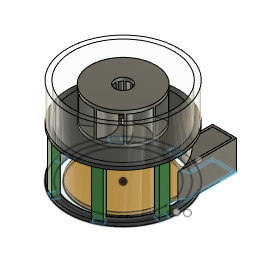
Impeller Design v6 (Autodesk Fusion 360 design; units mm, degrees)
Autodesk Fusion 360 part; units mm, degrees
sketch "Skizze1" plane through (0, 0, 0) normal (0, 0, 1) x (1, 0, 0)
  circle A0 centre (0, 0) radius 100
  circle A1 centre (0, 0) radius 25
  dimension "d1" = 200
  dimension "d2" = 50
  constraint coincident A0.centre A1.centre
  constraint concentric A0 A1
  measures "d1" diameter of A0
  measures "d2" diameter of A1
extrude "Extrusion1" add sketch "Skizze1" along normal blind 10 makes body 1
sketch "Skizze2" plane through (0, 0, 10) normal (0, 0, 1) x (-1, 0, 0)
  circle A0 centre (0, 0) radius 25
  circle A1 centre (0, 0) radius 100
  arc A2 (-99.7406, 7.1978) -> (-24.9999, -0.0752) centre (-57.9964, 48.5089) ccw
  arc A3 (-99.9959, 0.9028) -> (-24.4169, -5.3679) centre (-57.9964, 48.5089) ccw
  arc A4 (-77.1816, -63.5845) -> (-15.254, -19.8069) centre (-75.6088, -0.1194) ccw
  arc A5 (-81.0324, -58.5982) -> (-19.1027, -16.1272) centre (-75.6088, -0.1194) ccw
  arc A6 (-18.2532, -98.32) -> (1.0464, -24.9781) centre (-57.8429, -48.6919) ccw
  arc A7 (-24.4082, -96.9755) -> (-4.2671, -24.6331) centre (-57.8429, -48.6919) ccw
  arc A8 (49.2161, -87.0504) -> (16.8572, -18.4617) centre (-13.0117, -74.4808) ccw
  arc A9 (43.6369, -89.9768) -> (12.5651, -21.6129) centre (-13.0117, -74.4808) ccw
  arc A10 (93.6566, -35.049) -> (24.7803, -3.3069) centre (37.9078, -65.4194) ccw
  arc A11 (91.2637, -40.877) -> (23.5179, -8.4798) centre (37.9078, -65.4194) ccw
  arc A12 (94.2742, 33.3522) -> (21.1085, 13.3953) centre (71.0898, -25.7475) ccw
  arc A13 (96.1873, 27.3496) -> (23.4665, 8.6211) centre (71.0898, -25.7475) ccw
  arc A14 (50.7798, 86.1476) -> (7.5597, 23.8296) centre (71.0082, 25.9719) ccw
  arc A15 (56.1038, 82.779) -> (12.4348, 21.6881) centre (71.0082, 25.9719) ccw
  arc A16 (-16.475, 98.6335) -> (-9.5263, 23.1138) centre (37.701, 65.5388) ccw
  arc A17 (-10.2314, 99.4752) -> (-4.4152, 24.607) centre (37.701, 65.5388) ccw
  arc A18 (-76.021, 64.9677) -> (-22.1549, 11.5828) centre (-13.2469, 74.4394) ccw
  arc A19 (-71.7791, 69.6259) -> (-19.1994, 16.012) centre (-13.2469, 74.4394) ccw
  dimension "d7" = 360
  constraint coincident A1 A2.start
  constraint coincident A0 A2.end
  constraint concentric A2 A3
  constraint coincident A0 A3.end
  constraint coincident A1 A3.start
copy_body "Körper kopieren/einfügen1" bodies 1 makes body 2
move_body "Verschieben1" bodies 2 to x (1, 0, 0) y (0, 1, 0) z (0, 0, 1) at (0, 0, 90)
extrude "Extrusion2" add sketch "Skizze2" along normal up to surface (80 mm away) contours A0 A1 A12 A13 | A0 A1 A10 A11 | A0 A1 A14 A15 | A0 A1 A8 A9 | A0 A1 A16 A17 | A0 A1 A6 A7 | A0 A1 A18 A19 | A0 A1 A4 A5 | A0 A1 A2 A3 bodies 1 2
ref_plane "Arbeitsebene1" through (0, 0, -790) normal (0, 0, -1) x (-1, 0, 0)
sketch "Skizze3" plane through (0, 0, -790) normal (0, 0, -1) x (1, 0, 0)
  circle A0 centre (0, 0) radius 150
  circle A1 centre (0, 0) radius 170
  circle A2 centre (0, 0) radius 130
  line L0 (-13.6205, -169.4535) -> (13.6205, -169.4535)
  line L1 (13.6205, -169.4535) -> (13.6205, -149.4354)
  line L2 (13.6205, -149.4354) -> (-13.6205, -149.4354)
  line L3 (-13.6205, -149.4354) -> (-13.6205, -169.4535)
  line L4 (148.7196, 19.9735) -> (168.2358, 24.428)
  line L5 (162.1741, 50.9859) -> (142.6579, 46.5315)
  line L6 (142.6579, 46.5315) -> (148.7196, 19.9735)
  line L7 (168.2358, 24.428) -> (162.1741, 50.9859)
  line L8 (77.1092, 128.7269) -> (85.7947, 146.7626)
  line L9 (61.2515, 158.582) -> (52.5659, 140.5463)
  line L10 (52.5659, 140.5463) -> (77.1092, 128.7269)
  line L11 (85.7947, 146.7626) -> (61.2515, 158.582)
  line L12 (-52.5659, 140.5463) -> (-61.2515, 158.582)
  line L13 (-85.7947, 146.7626) -> (-77.1092, 128.7269)
  line L14 (-77.1092, 128.7269) -> (-52.5659, 140.5463)
  line L15 (-61.2515, 158.582) -> (-85.7947, 146.7626)
  line L16 (-142.6579, 46.5315) -> (-162.1741, 50.9859)
  line L17 (-168.2358, 24.428) -> (-148.7196, 19.9735)
  line L18 (-148.7196, 19.9735) -> (-142.6579, 46.5315)
  line L19 (-162.1741, 50.9859) -> (-168.2358, 24.428)
  line L20 (-125.3255, -82.5225) -> (-140.9763, -95.0036)
  line L21 (-123.9918, -116.3014) -> (-108.341, -103.8204)
  line L22 (-108.341, -103.8204) -> (-125.3255, -82.5225)
  line L23 (-140.9763, -95.0036) -> (-123.9918, -116.3014)
  line L24 (163, 0) -> (163, -1.523)
  line L25 (148.7196, -200) -> (75, -200)
  line L26 (75, -200) -> (75, -129.9038)
  line L27 (148.7196, 19.9735) -> (148.7196, 19.5574)
  line L28 (148.7196, -19.5574) -> (148.7196, -200)
  line L29 (141.7196, -49.1484) -> (141.7196, -193)
  line L30 (141.7196, -193) -> (82, -193)
  line L31 (82, -193) -> (82, -125.6025)
  arc A3 (82, -125.6025) -> (47.8354, -120.8792) centre (57.8269, -174.5291) ccw
  arc A4 (129.6641, -9.3398) -> (141.7196, -49.1484) centre (182.9727, -14.9257) ccw
  dimension "d11" = 300
  dimension "d12" = 20
  dimension "d13" = -20
  dimension "d15" = 360
  constraint coincident A0.centre A1.centre
  constraint perpendicular L0 L1
  constraint parallel L0 L2
  constraint parallel L1 L3
  constraint coincident A1 L0.end
  constraint horizontal L0
  constraint coincident A1 L0.start
  constraint vertical L27
  constraint perpendicular L25 L27
  constraint perpendicular L25 L26
  constraint collinear L27 L28
  constraint coincident A0 L27.end
  constraint parallel L28 L29
  constraint parallel L25 L30
  constraint parallel L26 L31
  constraint coincident A0 L29.start
  constraint coincident A0 L31.end
  constraint coincident A0 L26.end
  constraint coincident A2 A3.end
  constraint coincident A2 A4.start
  constraint coincident A0 L28.start
  measures "d11" diameter of A0
ref_plane "Arbeitsebene2" through (0, 0, -640) normal (0, 0, -1) x (1, 0, 0)
sketch "Skizze4" plane through (0, 0, -640) normal (0, 0, -1) x (1, 0, 0)
  circle A0 centre (0, 0) radius 170
  dimension "d17" = 340
  constraint coincident A0.centre origin
  measures "d17" diameter of A0
extrude "Extrusion3" add sketch "Skizze3" against normal blind 10 separate body contours A0 A1 L4 L27 L28 | A0 L6 L27 | A0 A1 L28 L29 | A0 L4 L5 L6 L7 | A0 A1 L29 L31 | A0 A1 L5 L6 L8 L10 | A1 L7 | A0 A1 L26 L31 | A2 A4 | A2 A4 | A0 L8 L9 L10 L11 | A0 A1 L1 L2 L26 | A0 A1 L9 L10 L12 L14 | A1 L11 | A0 L0 L1 L2 L3 | A0 L12 L13 L14 L15 | A0 A1 L2 L3 L21 L22 | A1 L0 | A0 A1 L13 L14 L16 L18 | A1 L15 | A0 L20 L21 L22 L23 | A0 L16 L17 L18 L19 | A0 A1 L17 L18 L20 L22 | A1 L23 | A1 L19 makes body 3 at (-159.6244, 32.6006, -790) makes body 4 at (49.7376, 0.9653, -790)
extrude "Extrusion4" add sketch "Skizze4" against normal blind 10 separate body makes body 5
extrude "Extrusion5" add sketch "Skizze3" against normal up to surface (150 mm away) separate body contours A0 L4 L5 L6 L7 | A0 L8 L9 L10 L11 | A0 L0 L1 L2 L3 | A0 L12 L13 L14 L15 | A0 L20 L21 L22 L23 | A0 L16 L17 L18 L19 makes body 6 at (166.2152, -33.2806, -690) makes body 7 at (-164.1946, -42.1333, -740) makes body 8 at (77.6137, -150.7024, -740) makes body 9 at (-4.5402, 169.4535, -740) makes body 10 at (-135.3148, 102.1029, -740) makes body 11 at (-69.4326, -154.6422, -740)
extrude "Extrusion6" add sketch "Skizze3" against normal blind 10 separate body contours A1 L29 L30 L31 makes body 12
copy_body "Körper kopieren/einfügen2" bodies 12 makes body 13
move_body "Verschieben2" bodies 13 to x (1, 0, 0) y (0, 1, 0) z (0, 0, 1) at (0, 0, 80)
extrude "Extrusion9" add sketch "Skizze3" against normal blind 10 separate body contours A0 A2 L2 L6 L10 L14 L18 L22 A3 A4 | A0 L6 | A0 A2 A3 A4 | A0 L10 | A0 L2 | A0 L14 | A0 L22 | A0 L18 makes body 14
sketch "Skizze6" plane through (0, 0, -780) normal (0, 0, 1) x (-1, 0, 0)
  circle A0 centre (0, 0) radius 150
  circle A1 centre (0, 0) radius 150
  circle A2 centre (0, 0) radius 148
  circle A3 centre (0, 0) radius 170
  dimension "d35" = -2
  constraint coincident A0.centre A1.centre
extrude "Extrusion10" add sketch "Skizze6" along normal up to surface (140 mm away) separate body contours A0 A1 makes body 15
sketch "Skizze7" plane through (0, 0, -630) normal (0, 0, 1) x (-1, 0, 0)
  circle A0 centre (0, 0) radius 170
  circle A1 centre (0, 0) radius 25
  circle A2 centre (0, 0) radius 155
  dimension "d38" = 50
  dimension "d41" = -15
  constraint coincident A0.centre A1.centre
  measures "d38" diameter of A1
extrude "Extrusion11" cut sketch "Skizze7" against normal blind 10 contours A1 bodies 5
move_body "Verschieben3" bodies 1 to x (1, 0, 0) y (0, 1, 0) z (0, 0, 1) at (0, 0, -630)
extrude "Extrusion12" add sketch "Skizze7" along normal blind 110 separate body contours A0 makes body 16
delete_body "Körper entfernen1" bodies 14
extrude "Extrusion13" add sketch "Skizze3" against normal blind 10 separate body contours A0 A2 A3 A4 makes body 17
combine "Kombinieren1" operation add target body 4 tool bodies 17
delete_body "Körper entfernen2" bodies 13
extrude "Extrusion14" add sketch "Skizze3" against normal blind 90 separate body contours A0 A1 L28 L29 | A1 L25 L26 L28 L29 L30 L31 | A0 A1 L26 L31 makes body 18
sketch "Skizze8" plane through (0, 200, 0) normal (0, 1, 0) x (-1, 0, 0)
  line L0 (-148.7196, -790) -> (-75, -790)
  line L1 (-75, -790) -> (-75, -700)
  line L2 (-75, -700) -> (-148.7196, -700)
  line L3 (-148.7196, -700) -> (-148.7196, -790)
  line L4 (-138.7196, -780) -> (-85, -780)
  line L5 (-85, -780) -> (-85, -710)
  line L6 (-85, -710) -> (-138.7196, -710)
  line L7 (-138.7196, -710) -> (-138.7196, -780)
  dimension "d48" = -10
extrude "Extrusion15" cut sketch "Skizze8" against normal blind 170 contours L4 L5 L6 L7 bodies 15 18
copy_body "Körper kopieren/einfügen3" bodies 12 makes body 19
copy_body "Körper kopieren/einfügen4" bodies 12 makes body 20
move_body "Verschieben4" bodies 20 to x (1, 0, 0) y (0, 1, 0) z (0, 0, 1) at (0, 0, 80)
move_face "Flächen versetzen1" offset 20 1 faces at (137.8322, 99.5102, -703.3333) on bodies 20
named bodies: "Impeller", "Top", "Support 1", "Support 2", "Support 3", "Support 4", "Support 5", "Support 6", "Bottom", "Dustbed", "Dustbed Connector", "Acryl shield Separator", "Acryl shield Impeller"
